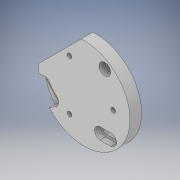
# Autodesk Inventor part: Encoder Mount Base
Saved by Autodesk Inventor 2018 (Build 220112000, 112)
## iProperties
Created: 2018-03-20
Part Number: Encoder Mount Base
Material: Generic
Document SubType Name: Modeling
Designer: P301319
Density: 1 g/cm^3
Appearance: Default
Author: P301319
Autodesk Inventor part; units mm, degrees
ref_plane "YZ Plane" through (0, 0, 0) normal (1, 0, 0) x (0, 1, 0)
ref_plane "XZ Plane" through (0, 0, 0) normal (0, 1, 0) x (-1, 0, 0)
ref_plane "XY Plane" through (0, 0, 0) normal (0, 0, 1) x (1, 0, 0)
sketch "Sketch1" plane through (0, 0, 0) normal (0, 0, 1) x (1, 0, 0)
  arc A0 (-39.1074, 3.3431) -> (-3.3431, 39.1074) centre (0, 0) ccw
  line L0 (0, 0) -> (30.017, 0) construction
  line L1 (-39.1074, 3.3431) -> (-3.3431, 39.1074)
  line L2 (0, 0) -> (39.25, 0) construction
  circle A1 centre (22.8042, -22.8042) radius 3
  circle A2 centre (-26.9378, -17.7318) radius 3
  circle A3 centre (17.7318, 26.9378) radius 3
  dimension "d0" = 78.5
  dimension "d6" = 6
  dimension "d9" = 6
  dimension "d10" = 6
  constraints: 6 end point, 4 centre point, 2 horizontal, 2 point on circle, 1 coincident
  measures "d0" diameter of A0
  measures "d6" diameter of A1
  measures "d9" diameter of A2
  measures "d10" diameter of A3
extrude "Extrusion1" add sketch "Sketch1" along normal blind 10
sketch "Sketch2" plane through (0, 0, 10) normal (0, 0, 1) x (1, 0, 0)
  circle A0 centre (17.7318, 26.9378) radius 3 projected
  circle A1 centre (17.7318, 26.9378) radius 5
  circle A2 centre (22.8042, -22.8042) radius 3 projected
  circle A3 centre (22.8042, -22.8042) radius 5
  circle A4 centre (-26.9378, -17.7318) radius 3 projected
  circle A5 centre (-26.9378, -17.7318) radius 5
  point P0 (0, 0)
  dimension "d13" = 10
  dimension "d14" = 10
  dimension "d15" = 10
  constraints: 3 centre point, 3 coincident
  measures "d13" diameter of A1
  measures "d14" diameter of A3
  measures "d15" diameter of A5
extrude "Extrusion2" cut sketch "Sketch2" against normal blind 5 contours A1
extrude "Extrusion3" cut sketch "Sketch2" against normal blind 5 contours A5
extrude "Extrusion4" cut sketch "Sketch2" against normal blind 5 contours A3
sketch "Sketch3" plane through (0, 0, 10) normal (0, 0, 1) x (1, 0, 0)
  line L0 (0, 0) -> (25, 0) construction
  circle A0 centre (-12.5, -21.6506) radius 2
  arc A1 (-39.1074, 3.3431) -> (-3.3431, 39.1074) centre (0, 0) ccw projected
  circle A2 centre (25, 0) radius 2
  circle A3 centre (-12.5, 21.6506) radius 2
  dimension "d24" = 4
  dimension "d27" = 360
  constraints: 3 centre point, 2 end point, 1 horizontal, 7 other
  measures "d24" diameter of A0
extrude "Extrusion5" cut sketch "Sketch3" against normal through all contours A0
extrude "Extrusion6" cut sketch "Sketch3" against normal through all contours A2
extrude "Extrusion7" cut sketch "Sketch3" against normal through all contours A3
sketch "Sketch4" plane through (0, 0, 0) normal (0, 0, -1) x (-1, 0, 0)
  circle A0 centre (12.5, 21.6506) radius 2 projected
  circle A1 centre (12.5, 21.6506) radius 4
  circle A2 centre (-25, 0) radius 2 projected
  circle A3 centre (-25, 0) radius 4
  circle A4 centre (12.5, -21.6506) radius 2 projected
  circle A5 centre (12.5, -21.6506) radius 4
  point P0 (0, 0)
  dimension "d35" = 8
  dimension "d36" = 8
  dimension "d37" = 8
  constraints: 3 centre point, 3 coincident
  measures "d35" diameter of A1
  measures "d36" diameter of A3
  measures "d37" diameter of A5
extrude "Extrusion8" cut sketch "Sketch4" against normal blind 5 contours A1
extrude "Extrusion9" cut sketch "Sketch4" against normal blind 5 contours A5
extrude "Extrusion10" cut sketch "Sketch4" against normal blind 5 contours A3
sketch "Sketch5" plane through (0, 0, 10) normal (0, 0, 1) x (1, 0, 0)
  circle A0 centre (17.7318, 26.9378) radius 3 projected
  circle A1 centre (22.8042, -22.8042) radius 3 projected
  circle A2 centre (-26.9378, -17.7318) radius 5 projected
  arc A3 (-39.1074, 3.3431) -> (-3.3431, 39.1074) centre (0, 0) ccw projected
  arc A4 (-30.0025, -6.3107) -> (-23.4023, -14.1962) centre (17.7318, 26.9378) ccw
  line L0 (-38.9658, -4.7151) -> (-34.7002, -4.204)
  line L1 (-24.2556, -21.9514) -> (-29.8381, -25.5)
  circle A5 centre (-26.9378, -17.7318) radius 5 projected
  arc A6 (-30.0025, -6.3107) -> (-34.7002, -4.204) centre (-34.1053, -9.1685) ccw
  arc A7 (12.2473, -17.7267) -> (22.2969, -17.83) centre (17.7318, 26.9378) ccw
  arc A8 (11.0285, -27.6521) -> (23.3114, -27.7784) centre (17.7318, 26.9378) ccw
  circle A9 centre (22.8042, -22.8042) radius 5 projected
  constraints: 14 point on circle, 4 centre point, 4 end point, 2 coincident, 2 tangent
extrude "Extrusion11" cut sketch "Sketch5" against normal blind 5 contours A2 L1 A3 L0 A6 A4
sketch "Sketch6" plane through (0, 0, 5) normal (0, 0, 1) x (1, 0, 0)
  circle A0 centre (17.7318, 26.9378) radius 3 projected
  circle A1 centre (22.8042, -22.8042) radius 3 projected
  circle A2 centre (-26.9378, -17.7318) radius 3 projected
  arc A3 (12.0035, -19.7118) -> (22.4998, -19.8197) centre (17.7318, 26.9378) ccw
  arc A4 (11.2723, -25.6671) -> (23.1085, -25.7887) centre (17.7318, 26.9378) ccw
  arc A5 (12.2473, -17.7267) -> (11.0285, -27.6521) centre (11.6379, -22.6894) ccw projected
  arc A6 (12.0035, -19.7118) -> (11.2723, -25.6671) centre (11.6379, -22.6894) ccw
  arc A7 (-31.6436, -7.4538) -> (-24.8165, -15.6104) centre (17.7318, 26.9378) ccw
  arc A8 (-36.567, -10.8831) -> (-29.0592, -19.8531) centre (17.7318, 26.9378) ccw
  arc A9 (-30.0025, -6.3107) -> (-34.7002, -4.204) centre (-34.1053, -9.1685) ccw projected
  arc A10 (-31.6436, -7.4538) -> (-36.567, -10.8831) centre (-34.1053, -9.1685) ccw
  point P0 (0, 0)
  dimension "d69" = 106
  dimension "d70" = 6
  dimension "d71" = 6
  constraints: 16 point on circle, 6 centre point, 5 coincident, 2 tangent
  measures "d69" diameter of A4
  measures "d70" radial gap between concentric circles of A7 A8
  measures "d71" diameter of A10
extrude "Extrusion14" cut sketch "Sketch6" against normal blind 5 contours A2 | A2 A8 A10 A7
sketch "Sketch7" plane through (0, 0, 10) normal (0, 0, 1) x (1, 0, 0)
  line L0 (-3.3431, 39.1074) -> (-39.1074, 3.3431) projected
  arc A0 (-29.8381, -25.5) -> (-3.3431, 39.1074) centre (0, 0) ccw projected
  line L1 (-2.5781, 39.1652) -> (-39.1652, 2.5781)
  line L2 (-2.5781, 39.1652) -> (49.1639, 39.1652) construction
  arc A1 (-39.1074, 3.3431) -> (-38.9658, -4.7151) centre (0, 0) ccw projected
  dimension "d77" = 135
  constraints: 4 end point, 2 point on circle, 1 equal length, 1 horizontal
  measures "d77" angle of L1 L2
extrude "Extrusion15" cut sketch "Sketch7" against normal blind 10
sketch "Sketch8" plane through (0, 0, 10) normal (0, 0, 1) x (1, 0, 0)
  circle A0 centre (17.7318, 26.9378) radius 3 projected
  line L0 (17.7318, 26.9378) -> (67.7318, 26.9378) construction
  circle A1 centre (22.8042, -22.8042) radius 3 projected
  arc A2 (14.342, -17.9343) -> (13.5888, -27.9059) centre (13.9654, -22.9201) ccw
  arc A3 (14.342, -17.9343) -> (22.2969, -17.83) centre (17.7318, 26.9378) ccw
  arc A4 (13.5888, -27.9059) -> (23.3114, -27.7784) centre (17.7318, 26.9378) ccw
  circle A5 centre (22.8042, -22.8042) radius 5 projected
  point P0 (0, 0)
  dimension "d84" = 10
  dimension "d87" = 10
  constraints: 8 point on circle, 3 centre point, 2 end point, 1 coincident, 1 horizontal
  measures "d84" diameter of A2
  measures "d87" radial gap between concentric circles of A3 A4
extrude "Extrusion16" cut sketch "Sketch8" against normal blind 5 contours A3 A5 A4 A2 | A5
sketch "Sketch9" plane through (0, 0, 5) normal (0, 0, 1) x (1, 0, 0)
  arc A0 (14.342, -17.9343) -> (13.5888, -27.9059) centre (13.9654, -22.9201) ccw projected
  arc A1 (14.1914, -19.9286) -> (13.7394, -25.9116) centre (13.9654, -22.9201) ccw
  circle A2 centre (17.7318, 26.9378) radius 3 projected
  circle A3 centre (22.8042, -22.8042) radius 3 projected
  arc A4 (14.1914, -19.9286) -> (22.4998, -19.8197) centre (17.7318, 26.9378) ccw
  arc A5 (13.7394, -25.9116) -> (23.1085, -25.7887) centre (17.7318, 26.9378) ccw
  point P0 (0, 0)
  dimension "d90" = 6
  dimension "d92" = 6
  constraints: 8 point on circle, 3 centre point, 2 coincident
  measures "d90" diameter of A1
  measures "d92" radial gap between concentric circles of A4 A5
extrude "Extrusion17" cut sketch "Sketch9" against normal blind 5 contours A4 A3 A5 A1
body "Solid1"
